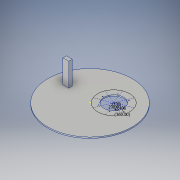
# Autodesk Inventor part: 55K stage
Saved by Autodesk Inventor 2018 (Build 220112000, 112)
## iProperties
Created: 2018-10-14
Part Number: 55K stage
Material: Aluminum 6061
Document SubType Name: Modeling
Designer: freyja
Density: 2.7 g/cm^3
Appearance: Aluminum - Flat
Mass: 2661.5 g
Surface Area: 3217.19 cm^2
Volume: 985.742 cm^3
Author: freyja
Autodesk Inventor part; units mm, degrees
ref_plane "YZ Plane" through (0, 0, 0) normal (1, 0, 0) x (0, 1, 0)
ref_plane "XZ Plane" through (0, 0, 0) normal (0, 1, 0) x (-1, 0, 0)
ref_plane "XY Plane" through (0, 0, 0) normal (0, 0, 1) x (1, 0, 0)
sketch "Sketch1" plane through (0, 0, 0) normal (0, 1, 0) x (-1, 0, 0)
  circle A0 centre (0, 0) radius 228.6
  dimension "d0" = 457.2
  constraints: 1 centre point, 1 coincident
  measures "d0" diameter of A0
extrude "Extrusion1" add sketch "Sketch1" along normal blind 6.35
sketch "Sketch2" plane through (0, 6.35, 0) normal (0, 1, 0) x (1, 0, 0)
  line L0 (0, 0) -> (64.6578, 64.6578) construction
  line L1 (0, 0) -> (91.44, 0) construction
  circle A0 centre (64.6578, 64.6578) radius 53.34
  circle A1 centre (64.6578, 64.6578) radius 46.99 construction
  dimension "d3" = 91.44
  dimension "d4" = 45
  dimension "d5" = 106.68
  dimension "d6" = 93.98
  constraints: 4 end point, 2 centre point, 2 coincident, 1 equal length, 1 horizontal, 1 point on line
  measures "d3" distance of L0.start L0.end
  measures "d4" angle of L1 L0
  measures "d5" diameter of A0
  measures "d6" diameter of A1
extrude "Extrusion2" cut sketch "Sketch2" against normal up to surface (6.35 mm away)
sketch "Sketch4" plane through (0, 6.35, 0) normal (0, 1, 0) x (1, 0, 0)
  circle A0 centre (64.6578, 64.6578) radius 53.34 projected
  line L0 (64.6578, 64.6578) -> (124.9828, 64.6578)
  line L1 (64.6578, 64.6578) -> (124.9828, 64.6578) construction
  line L2 (64.6578, 64.6578) -> (94.8203, 116.9008)
  line L3 (64.6578, 64.6578) -> (34.4953, 116.9008)
  line L4 (64.6578, 64.6578) -> (4.3328, 64.6578)
  line L5 (64.6578, 64.6578) -> (34.4953, 12.4149)
  line L6 (64.6578, 64.6578) -> (94.8203, 12.4149)
  point P0 (0, 0)
  dimension "d22" = 60.325
  dimension "d23" = 0
  dimension "d26" = 360
  constraints: 14 end point, 2 coincident, 1 collinear, 1 horizontal, 17 other
  measures "d22" distance of L0.start L0.end
  measures "d23" distance between parallel lines of L1 L0
hole "Hole2" at (124.9828, 6.35, -64.6578) at (94.8203, 6.35, -116.9008) at (34.4953, 6.35, -116.9008) at (4.3328, 6.35, -64.6578) at (34.4953, 6.35, -12.4149) at (94.8203, 6.35, -12.4149) direction (0, -1, 0) diameter 4.1402 end up to face face through (-97.7389, 0, 99.5327) facing (0, -1, 0)
sketch "Sketch5" plane through (0, 6.35, 0) normal (0, 1, 0) x (1, 0, 0)
  line L0 (-158.75, 30.1625) -> (-127, 30.1625)
  line L1 (-127, 30.1625) -> (-127, 11.1125)
  line L2 (-127, 11.1125) -> (-158.75, 11.1125)
  line L3 (-158.75, 11.1125) -> (-158.75, 30.1625)
  point P0 (0, 0)
  constraints: 8 end point, 2 parallel, 1 horizontal, 1 perpendicular
extrude "Extrusion3" add sketch "Sketch5" along normal blind 127
sketch "Sketch6" plane through (0, 6.35, 0) normal (0, 1, 0) x (1, 0, 0)
  line L0 (64.6578, 64.6578) -> (144.4441, 31.6093) construction
  line L1 (64.6578, 64.6578) -> (144.4441, 97.7064) construction
  line L2 (64.6578, 64.6578) -> (97.7064, 144.4441) construction
  line L3 (64.6578, 64.6578) -> (31.6093, 144.4441) construction
  line L4 (64.6578, 64.6578) -> (-15.1284, 97.7064) construction
  line L5 (64.6578, 64.6578) -> (-15.1284, 31.6093) construction
  line L6 (64.6578, 64.6578) -> (31.6093, -15.1284) construction
  line L7 (64.6578, 64.6578) -> (97.7064, -15.1284) construction
  line L8 (64.6578, 64.6578) -> (111.5909, 45.2175) construction
  line L9 (64.6578, 64.6578) -> (115.4578, 64.6578) construction
  point P0 (0, 0)
  dimension "d37" = 86.36
  dimension "d38" = 360
  dimension "d39" = 50.8
  dimension "d40" = 22.5
  constraints: 20 end point, 2 coincident, 1 collinear, 1 equal length, 1 horizontal, 23 other
  measures "d37" distance of L0.start L0.end
  measures "d39" distance of L7.start L8.end
  measures "d40" angle of L8 L9
body "Solid1"
